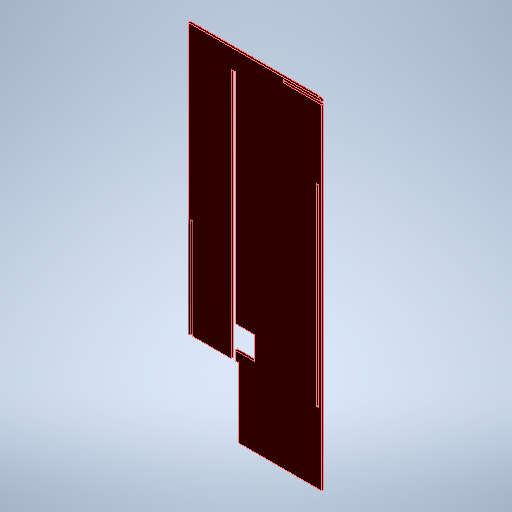
# Autodesk Inventor part: Finishing Sheets .1  ( Right )
Saved by Autodesk Inventor 2025.4 (Build 294407000, 407)
## iProperties
Created: 2026-04-04
Part Number: Finishing Sheets .1  ( Right )
Material: Generic
Document SubType Name: Sheet Metal
Designer: lenovo
Density: 1 g/cm^3
Sheet Metal Rule: Default_mm
Appearance: Default(1)
Author: lenovo
Autodesk Inventor part; units mm, degrees
ref_plane "YZ Plane" through (0, 0, 0) normal (1, 0, 0) x (0, 1, 0)
ref_plane "XZ Plane" through (0, 0, 0) normal (0, 1, 0) x (-1, 0, 0)
ref_plane "XY Plane" through (0, 0, 0) normal (0, 0, 1) x (1, 0, 0)
sketch "Sketch8" plane through (0, 0, 3) normal (0, 0, 1) x (1, 0, 0)
  line L0 (-83.75, -130) -> (-83.75, 220)
  line L1 (-83.75, 220) -> (-89.75, 220)
  line L2 (-89.75, 220) -> (-89.75, -130)
  line L3 (-89.75, -130) -> (-83.75, -130)
  line L4 (-83.75, -130) -> (-83.75, 220)
  line L5 (-86.75, -130) -> (-86.75, 0)
  line L6 (-86.75, 0) -> (-83.75, 0)
  point P0 (0, 0)
  dimension "d35" = 6
  measures "d35" distance of L3.end L2.end
sketch "Sketch1" plane through (0, 0, 0) normal (0, 0, 1) x (1, 0, 0)
  line L0 (-83.75, -220) -> (83.75, -220)
  line L1 (83.75, -220) -> (83.75, 220)
  line L2 (83.75, 220) -> (-83.75, 220)
  line L3 (-83.75, 220) -> (-83.75, -220)
  line L4 (-83.75, -220) -> (83.75, 220) construction
  line L5 (83.75, -220) -> (-83.75, 220) construction
  point P0 (0, 0)
  dimension "d0" = 440
  dimension "d1" = 167.5
  measures "d0" distance of L1.end L0.end
  measures "d1" distance of L1.end L2.end
extrude "Plate1" add sketch "Sketch1" along normal blind 3
sketch "Sketch3" plane through (0, 0, 3) normal (0, 0, 1) x (1, 0, 0)
  line L0 (-83.75, -220) -> (83.75, -220) projected
  line L1 (-83.75, -220) -> (-23.75, -220)
  line L2 (-23.75, -220) -> (-23.75, -130)
  line L3 (-23.75, -130) -> (-83.75, -130)
  line L4 (-83.75, -130) -> (-83.75, -220)
  point P0 (0, 0)
  dimension "d7" = 60
  dimension "d8" = 90
  constraints: 8 end point, 2 parallel, 1 horizontal, 1 perpendicular
  measures "d7" distance of L3.end L2.end
  measures "d8" distance of L2.end L1.end
extrude "Cut2" cut sketch "Sketch3" against normal blind 3
sketch "Sketch4" plane through (0, 0, 3) normal (0, 0, 1) x (1, 0, 0)
  line L0 (-83.75, 220) -> (-83.75, -130) projected
  line L1 (-28.75, -88) -> (-3.75, -88)
  line L2 (-3.75, -88) -> (-3.75, -118)
  line L3 (-3.75, -118) -> (-83.75, -118)
  line L4 (-83.75, -118) -> (-83.75, -93)
  line L5 (-83.75, -130) -> (-23.75, -130) projected
  line L6 (-28.75, -88) -> (-28.75, -118)
  point P0 (0, 0)
  dimension "d11" = 12
  dimension "d12" = 30
  dimension "d13" = 25
  dimension "d16" = 55
  constraints: 10 end point, 2 parallel, 2 perpendicular, 1 horizontal, 1 point on line
  measures "d11" distance between parallel lines of L5 L3
  measures "d12" distance of L1.end L2.end
  measures "d13" distance of L1.start L1.end
  measures "d16" distance between parallel lines of L6 L0
extrude "Cut3" cut sketch "Sketch4" against normal blind 3
sketch "Sketch5" plane through (0, 0, 3) normal (0, 0, 1) x (1, 0, 0)
  line L0 (-33.75, 195) -> (-28.75, 195)
  line L1 (-28.75, 195) -> (-28.75, -130)
  line L2 (-28.75, -130) -> (-33.75, -130)
  line L3 (-33.75, -130) -> (-33.75, 195)
  line L4 (-83.75, 220) -> (83.75, 220) projected
  line L5 (-83.75, -130) -> (-23.75, -130) projected
  line L6 (-83.75, -130) -> (-83.75, 220) projected
  point P0 (0, 0)
  point P1 (-31.25, -130)
  dimension "d17" = 25
  dimension "d18" = 5
  dimension "d19" = 50
  constraints: 8 end point, 2 parallel, 1 horizontal, 1 midpoint, 1 perpendicular, 1 point on line
  measures "d17" distance between parallel lines of L4 L0
  measures "d18" distance between parallel lines of L1 L3
  measures "d19" distance between parallel lines of L6 L3
extrude "Cut4" cut sketch "Sketch5" against normal blind 3
fillet "Corner Round1" radius 5 1 edges at (83.75, 220, 1.5)
sketch "Sketch6" plane through (0, 0, 3) normal (0, 0, 1) x (1, 0, 0)
  line L0 (83.75, 215) -> (83.75, -220) projected
  line L1 (83.75, 217) -> (33.75, 217)
  line L2 (33.75, 217) -> (33.75, 214)
  line L3 (33.75, 214) -> (83.75, 214)
  line L4 (83.75, 214) -> (83.75, 217)
  line L5 (-83.75, 220) -> (78.75, 220) projected
  point P0 (0, 0)
  point P1 (-78.75, 220)
  dimension "d24" = 50
  dimension "d25" = 3
  dimension "d26" = 3
  constraints: 8 end point, 2 parallel, 1 horizontal, 1 perpendicular, 1 point on line
  measures "d24" distance of L1.start L1.end
  measures "d25" distance between parallel lines of L5 L1
  measures "d26" distance between parallel lines of L1 L3
extrude "Cut5" cut sketch "Sketch6" against normal blind 3
sketch "Sketch7" plane through (0, 0, 3) normal (0, 0, 1) x (1, 0, 0)
  line L0 (76.75, 122) -> (79.75, 122)
  line L1 (79.75, 122) -> (79.75, -128)
  line L2 (79.75, -128) -> (76.75, -128)
  line L3 (76.75, -128) -> (76.75, 122)
  line L4 (83.75, 214) -> (83.75, -220) projected
  line L5 (83.75, -220) -> (-23.75, -220) projected
  point P0 (0, 0)
  dimension "d29" = 3
  dimension "d30" = 4
  dimension "d31" = 92
  dimension "d32" = 250
  constraints: 8 end point, 2 parallel, 1 horizontal, 1 perpendicular
  measures "d29" distance of L0.start L0.end
  measures "d30" distance between parallel lines of L4 L1
  measures "d31" distance between parallel lines of L5 L2
  measures "d32" distance of L0.end L1.end
extrude "Cut6" cut sketch "Sketch7" against normal blind 3
sheet face with bend "Face2" sketch "Sketch8" thickness 3 toward (0, 0, -1) bend radius 3 contours L6 L5 L3 L2 L1 L0
bend "Bend1"
equation "\"d9\" = Thickness"
equation "\"d14\" = Thickness"
equation "\"d20\" = Thickness"
equation "\"d27\" = Thickness"
equation "\"d33\" = Thickness"
equation "\"d2\" = Thickness"
equation "\"d36\" = BendRadius"
equation "\"d37\" = BendReliefWidth"
equation "\"d39\" = MinimumRemnant"
equation "\"d38\" = BendReliefDepth"
equation "\"d40\" = TransitionRadius"
equation "\"BendRadius\" = Thickness"
equation "\"BendReliefWidth\" = Thickness"
equation "\"BendReliefDepth\" = 0.5 * Thickness"
equation "\"CornerReliefSize\" = 4 * Thickness"
equation "\"MinimumRemnant\" = 2 * Thickness"
equation "\"TransitionRadius\" = BendRadius"
equation "\"JacobiRadiusSize\" = BendRadius"
equation "\"GapSize\" = Thickness"
equation "\"Thickness\" = 3"
body "Solid1"
